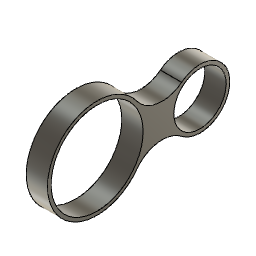
JRCNC0015 v7 (Autodesk Fusion 360 design; units mm, degrees)
Autodesk Fusion 360 part; units mm, degrees
note: some values were not read from the file. Set by a fixed rule: which sketch regions a step uses.
sketch "Sketch2" plane through (0, 0, 0) normal (1, 0, 0) x (0, 1, 0)
  circle A0 centre (73.75, 0) radius 21.29
  line L0 (0, 0) -> (147.5, 0) construction
  circle A1 centre (73.75, 0) radius 18.75
  line L1 (78.83, -20.32) -> (78.83, -17.78)
  circle A2 centre (0, 0) radius 35.49
  line L2 (35.49, 0) -> (52.46, 0)
  circle A3 centre (46.6735, 34.4155) radius 22.5
  circle A4 centre (46.6735, -34.4155) radius 22.5
  circle A5 centre (0, 0) radius 32.95
  dimension "d11" = 37.5
  dimension "d14" = 2.54
  dimension "d24" = 65.9
  dimension "d25" = 2.54
  dimension "d26" = 73.75
  dimension "d27" = 45
  constraint midpoint A0.centre L0
  constraint concentric A0 A1
  constraint vertical L1
  constraint coincident L0.start A2.centre
  constraint horizontal L0
  constraint coincident A2 L2.start
  constraint coincident L0 L2.start
  constraint coincident A0 L2.end
  constraint coincident L0 L2.end
  constraint tangent A0 A3
  constraint tangent A2 A3
  constraint tangent A2 A4
  constraint tangent A0 A4
  constraint equal A3 A4
  constraint concentric A2 A5
  measures "d11" diameter of A1
  measures "d14" distance of A0 A1
  measures "d24" diameter of A5
  measures "d25" distance of A2 A5
  measures "d26" distance of A0.centre L0.start
  measures "d27" diameter of A3
extrude "Extrude2" add sketch "Sketch2" along normal blind 15.24 contours A0 | A0 A2 L2 A3 | A0 A2 L2 A4 | A2
